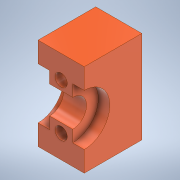
# Autodesk Inventor part: Print_Parts_A2
Saved by Autodesk Inventor 2020 (Build 240168000, 168)
## iProperties
Created: 2020-10-05
Part Number: Print_Parts_A2
Material: PC/ABS プラスチック
Document SubType Name: Modeling
Designer: kenta iguchi
Density: 0.357273 g/cm^3
Appearance: 滑らか - 淡いオレンジ
Author: kenta iguchi
Autodesk Inventor part; units mm, degrees
ref_plane "YZ Plane" through (0, 0, 0) normal (1, 0, 0) x (0, 1, 0)
ref_plane "XZ Plane" through (0, 0, 0) normal (0, 1, 0) x (-1, 0, 0)
ref_plane "XY Plane" through (0, 0, 0) normal (0, 0, 1) x (1, 0, 0)
sketch "スケッチ1" plane through (0, 0, 0) normal (0, 0, 1) x (1, 0, 0)
  line L0 (-10, -20) -> (10, -20)
  line L1 (10, -20) -> (10, 20)
  line L2 (10, 20) -> (-10, 20)
  line L3 (-10, 20) -> (-10, -20)
  line L4 (-10, -20) -> (10, 20) construction
  line L5 (10, -20) -> (-10, 20) construction
  point P0 (0, 0)
  dimension "d0" = 20
  dimension "d1" = 40
  constraints: 12 end point, 2 midpoint, 2 parallel, 1 horizontal, 1 perpendicular
  measures "d0" distance of L2.end L1.end
  measures "d1" distance of L1.end L0.end
extrude "押し出し1" add sketch "スケッチ1" along normal blind 25
sketch "スケッチ2" plane through (10, -20, 0) normal (1, 0, 0) x (0, 0, -1)
  circle A0 centre (-25, 20) radius 11.1
  line L0 (0, 40) -> (-25, 40) projected
  dimension "d4" = 22.2
  dimension "d7" = 20
  constraints: 1 centre point, 1 vertical alignment
  measures "d4" diameter of A0
  measures "d7" distance from line of L0 A0.centre
extrude "押し出し2" cut sketch "スケッチ2" against normal through all
sketch "スケッチ7" plane through (0, 0, 0) normal (1, 0, 0) x (0, 1, 0)
  arc A0 (-11.1, 25) -> (11.1, 25) centre (0, 25) ccw projected
  line L0 (20, 25) -> (11.1, 25) projected
  line L1 (20, 0) -> (20, 25) projected
  line L2 (20, 0) -> (-20, 0) projected
  line L3 (-20, 0) -> (-20, 25) projected
  line L4 (-11.1, 25) -> (-20, 25) projected
  circle A1 centre (0, 25) radius 6
  arc A2 (-11.1, 25) -> (11.1, 25) centre (0, 25) ccw projected
  line L5 (11.1, 25) -> (-11.1, 25)
  point P0 (0, 0)
  point P1 (-6, 25)
  point P2 (6, 25)
  dimension "d27" = 12
  constraints: 2 end point, 1 centre point, 1 coincident, 1 horizontal
  measures "d27" diameter of A1
extrude "押し出し5" add sketch "スケッチ7" along normal mid plane 10 contours L5 A1 A0
sketch "スケッチ5" plane through (0, 0, 25) normal (0, 0, 1) x (1, 0, 0)
  line L0 (10, 20) -> (-10, 20) projected
  line L1 (-10, -20) -> (10, -20) projected
  point P0 (0, 0)
  point P1 (0, 10)
  point P2 (0, -10)
  dimension "d18" = 10
  dimension "d19" = 10
  measures "d18" distance from line of point (0, 10) L0
  measures "d19" distance from line of point (0, -10) L1
hole "穴1" at (0, 10, 25) at (0, -10, 25) direction (0, 0, -1) diameter 5.3 depth 58
